Autodesk Fusion 360 part; units mm, degrees
note: some values were not read from the file. Set by a fixed rule: which sketch regions a step uses.
(part 4 of 4)
equation "SolarInput_Z_Size = 7.5 mm"
equation "d49 = SolarInput_X_Size"
equation "d50 = SolarInput_Y_Size"
equation "d51 = SolarInput_Y_Size - SolarInput_EdgeOverhang"
equation "SolarInput_EdgeOverhang = 3 mm"
equation "Antenna_PCB_Center_Offset = -4 mm"
equation "d54 = -Antenna_PCB_Center_Offset"
equation "d55 = PCB_Z_Size"
equation "d57 = BatteryHolder_Z_Size"
equation "d59 = SolarInput_Z_Size"
equation "d62 = BatteryHolder_Y_Size / 2"
equation "d64 = BatteryHolder_Y_Size / 2"
equation "d65 = PCB_Z_Size + 0.2 mm"
equation "d66 = USB_Jack_Z_Size"
equation "Screen_Z_Offset = 11 mm"
equation "d69 = Screen_Z_Offset"
equation "d70 = PCB_Z_Size"
equation "Screen_Display_Z_Size = 1.3 mm"
equation "Screen_Y_Size = 29.2 mm"
equation "d74 = Screen_PCB_X_Size"
equation "d75 = Screen_Y_Size"
equation "d76 = ( Screen_PCB_Y_Size - Screen_Y_Size ) / 2"
equation "d77 = Screen_Display_Z_Size"
equation "d80 = PCB_Bolt_Hole_Diameter"
equation "PCB_Bolt_Hole_Diameter = 2.1 mm"
equation "Enclosure_Wall_Thickness = 2 mm"
equation "PCB_Bottom_Z_Clearance = 3 mm"
equation "d85 = -PCB_Bottom_Z_Clearance"
equation "PCB_Horizontal_Clearance = 1 mm"
equation "d87 = PCB_Horizontal_Clearance"
equation "d88 = PCB_Horizontal_Clearance + Enclosure_Wall_Thickness"
equation "d89 = -Enclosure_Wall_Thickness"
equation "Cutout_Clearance = 1 mm"
equation "d102 = Cutout_Clearance"
equation "USB_C_Plug_X_Size = 14 mm"
equation "USB_C_Plug_Y_Size = 10 mm"
equation "d107 = USB_C_Plug_X_Size"
equation "d108 = USB_C_Plug_Y_Size"
equation "d112 = d111"
equation "d113 = Enclosure_Wall_Thickness"
equation "Battery_Ceiling_Clearance = 2 mm"
equation "d117 = -Battery_Ceiling_Clearance"
equation "d120 = Enclosure_Wall_Thickness"
equation "Antenna_Hole_Diameter = 10 mm"
equation "Antenna_PCB_Center_Z_Offset = 6.5 mm"
equation "d124 = Antenna_PCB_Center_Z_Offset + PCB_Z_Size"
equation "d126 = Antenna_Hole_Diameter"
equation "Enclosure_Bolt_Flange_Diameter = 6 mm"
equation "Enclosure_Chamfer = 1 mm"
equation "Heatset_Insert_Hole_Size = 3 mm"
equation "PCB_Corner_Radius = 2.5 mm"
equation "d167 = PCB_Corner_Radius"
equation "d168 = PCB_Corner_Radius"
equation "d169 = PCB_Corner_Radius"
equation "d170 = PCB_Corner_Radius"
equation "d171 = PCB_Corner_Radius"
equation "d172 = PCB_Corner_Radius"
equation "d173 = PCB_Corner_Radius"
equation "d174 = PCB_Corner_Radius"
equation "d175 = PCB_Corner_Radius"
equation "d176 = PCB_Corner_Radius"
equation "d177 = PCB_Corner_Radius"
equation "d178 = PCB_Corner_Radius"
equation "PCB_Bolt_Seat_Diameter = 6 mm"
equation "d192 = PCB_Horizontal_Clearance"
equation "d193 = PCB_Bolt_Seat_Diameter"
equation "d194 = PCB_Bolt_Seat_Diameter"
equation "d195 = PCB_Bolt_Seat_Diameter"
equation "d196 = PCB_Bolt_Seat_Diameter"
equation "d199 = PCB_Bottom_Z_Clearance"
equation "d201 = PCB_Bottom_Z_Clearance + Enclosure_Wall_Thickness - 1 mm"
equation "d202 = PCB_Bolt_Hole_Diameter"
equation "Bolt_Inset_Distance = 3.5 mm"
equation "d205 = -Bolt_Inset_Distance"
equation "d210 = Enclosure_Filet_Radius"
equation "Enclosure_Filet_Radius = 2 mm"
equation "d228 = Enclosure_Filet_Radius"
equation "d230 = Enclosure_Filet_Radius - 0.1 mm"
equation "d231 = Enclosure_Wall_Thickness - 0.5 mm"
